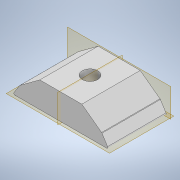
# Autodesk Inventor part: tripodSchwalbenschanz
Saved by Autodesk Inventor 2021 (Build 250183000, 183)
## iProperties
Created: 2020-07-08
Part Number: tripodSchwalbenschanz
Material: Generisch
Document SubType Name: Modeling
Designer: marvi
Density: 1 g/cm^3
Appearance: Vorgabe
Author: marvi
Autodesk Inventor part; units mm, degrees
sketch "Skizze1" plane through (0, 0, 0) normal (0, 0, 1) x (1, 0, 0)
  line L0 (-9, 4.8) -> (-9, 11)
  line L1 (-9, 11) -> (0, 11)
  line L2 (0, 13.225) -> (0, -2.3499) projected
  line L3 (0, 0) -> (-19.5979, 0)
  line L4 (-20.0219, 0.765) -> (-17.6469, 4.565)
  line L5 (-17.2229, 4.8) -> (-9, 4.8)
  arc A0 (-20.0219, 0.765) -> (-19.5979, 0) centre (-19.5979, 0.5) ccw
  arc A1 (-17.2229, 4.8) -> (-17.6469, 4.565) centre (-17.2229, 4.3) ccw
  line L6 (9, 4.8) -> (9, 11)
  line L7 (9, 11) -> (0, 11)
  line L8 (0, 0) -> (19.5979, 0)
  line L9 (20.0219, 0.765) -> (17.6469, 4.565)
  line L10 (17.2229, 4.8) -> (9, 4.8)
  arc A2 (19.5979, 0) -> (20.0219, 0.765) centre (19.5979, 0.5) ccw
  arc A3 (17.6469, 4.565) -> (17.2229, 4.8) centre (17.2229, 4.3) ccw
  line L11 (9, 11) -> (17.4653, 4.7373)
  line L12 (-9, 11) -> (-17.4653, 4.7373)
  point P0 (-20.5, 0)
  point P1 (20.5, 0)
  dimension "d5" = 6.2
  dimension "d6" = 9
  dimension "d9" = 20.5
  dimension "d11" = 0.5
  dimension "d12" = 0.5
  constraints: 24 end point, 10 horizontal alignment, 9 point on circle, 4 centre point, 4 point on line, 4 tangent, 2 equal radius, 2 horizontal, 1 perpendicular, 1 vertical, 1 other
  measures "d5" distance of L0.start L0.end
  measures "d6" distance of the line from the sketch origin of L0
  measures "d9" distance of L3.start point (-20.5, 0)
  measures "d11" radius of A0
  measures "d12" radius of A1
extrude "Extrusion1" add sketch "Skizze1" along normal blind 25
sketch "Skizze2" plane through (-19.5979, 0, 0) normal (0, -1, 0) x (1, 0, 0)
  line L0 (0, 0) -> (39.1958, 0) projected
  line L1 (39.1958, 0) -> (39.1958, 25) projected
  line L2 (0, 25) -> (39.1958, 25) projected
  line L3 (0, 0) -> (0, 25) projected
  point P0 (19.5979, 0)
  point P1 (19.5979, 12.5)
hole "Bohrung1" at (0, 0, 12.5) direction (0, 1, 0) diameter 6.6 end through all counterbore diameter 15 counterbore depth 6
